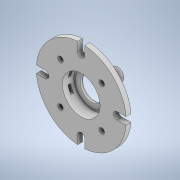
# Autodesk Inventor part: součást 4
Saved by Autodesk Inventor 2022 (Build 260153000, 153)
## iProperties
Created: 2022-03-28
Part Number: součást 4
Material: Všeobecné
Document SubType Name: Modeling
Designer: 27262
Density: 1 g/cm^3
Appearance: Výchozí
Author: 27262
Autodesk Inventor part; units mm, degrees
ref_plane "YZ Plane" through (0, 0, 0) normal (1, 0, 0) x (0, 1, 0)
ref_plane "XZ Plane" through (0, 0, 0) normal (0, 1, 0) x (-1, 0, 0)
ref_plane "XY Plane" through (0, 0, 0) normal (0, 0, 1) x (1, 0, 0)
sketch "Náčrt1" plane through (0, 0, 0) normal (1, 0, 0) x (0, 1, 0)
  line L0 (42, 0) -> (100, 0)
  line L1 (100, 0) -> (100, -11)
  line L2 (100, -11) -> (52, -11)
  line L3 (52, -11) -> (52, -39)
  line L4 (52, -39) -> (42.5, -39)
  line L5 (42.5, -39) -> (42.5, -30)
  line L6 (42.5, -30) -> (26.7321, -30)
  line L7 (26.7321, -30) -> (25, -27)
  line L8 (25, -27) -> (25, -23)
  line L9 (25, -23) -> (36, -23)
  line L10 (36, -23) -> (36, -25.5)
  line L11 (36, -25.5) -> (42, -25.5)
  line L12 (42, -25.5) -> (42, 0)
  line L13 (0, 0) -> (0, -39) construction
  dimension "d0" = 200
  dimension "d1" = 50
  dimension "d2" = 72
  dimension "d3" = 84
  dimension "d4" = 85
  dimension "d5" = 104
  dimension "d6" = 39
  dimension "d7" = 11
  dimension "d8" = 30
  dimension "d9" = 25.5
  dimension "d10" = 23
  dimension "d11" = 4
  dimension "d12" = 30
  constraints: 28 end point, 9 perpendicular, 2 horizontal alignment, 2 vertical, 1 horizontal, 1 parallel
  measures "d0" diameter of L1 L13
  measures "d1" diameter of L8 L13
  measures "d2" diameter of L10 L13
  measures "d3" diameter of L12 L13
  measures "d4" diameter of L5 L13
  measures "d5" diameter of L3 L13
  measures "d6" distance between parallel lines of L0 L4
  measures "d7" distance of L0.end L1.end
  measures "d8" distance between parallel lines of L0 L6
  measures "d9" distance between parallel lines of L0 L11
  measures "d10" distance between parallel lines of L0 L9
  measures "d11" distance of L7.end L8.end
  measures "d12" angle of L7 L8
revolve "Rotace1" add sketch "Náčrt1" angle 360 about axis through (0, 0, 0) along (0, 0, -1)
sketch "Náčrt2" plane through (0, 0, -11) normal (0, 0, -1) x (-1, 0, 0)
  circle A0 centre (0, 0) radius 100 projected
  line L0 (-100, 0) -> (-80, 0) construction
  line L1 (-100, -8) -> (-80, -8)
  line L2 (-80, 8) -> (-100, 8)
  arc A1 (-100, 8) -> (-100, -8) centre (-100, 0) ccw
  arc A2 (-80, -8) -> (-80, 8) centre (-80, 0) ccw
  circle A3 centre (0, 0) radius 52 projected
  line L3 (8, -100) -> (8, -80)
  arc A4 (-8, -100) -> (8, -100) centre (0, -100) ccw
  line L4 (-8, -80) -> (-8, -100)
  arc A5 (8, -80) -> (-8, -80) centre (0, -80) ccw
  line L5 (100, 8) -> (80, 8)
  arc A6 (100, -8) -> (100, 8) centre (100, 0) ccw
  line L6 (80, -8) -> (100, -8)
  arc A7 (80, 8) -> (80, -8) centre (80, 0) ccw
  line L7 (-8, 100) -> (-8, 80)
  arc A8 (8, 100) -> (-8, 100) centre (0, 100) ccw
  line L8 (8, 80) -> (8, 100)
  arc A9 (-8, 80) -> (8, 80) centre (0, 80) ccw
  point P0 (-90, 0)
  dimension "d14" = 16
  dimension "d15" = 80
  dimension "d18" = 360
  constraints: 20 end point, 16 point on circle, 8 centre point, 4 tangent, 2 horizontal alignment, 1 horizontal, 1 midpoint, 1 parallel, 42 other
  measures "d14" diameter of A2
  measures "d15" distance of A3.centre L0.end
extrude "Vysunutí1" cut sketch "Náčrt2" against normal through all contours A0 L6 A7 L5 | A0 L5 A6 L6 | L8 A9 L7 A0 | A0 L7 A8 L8 | L3 A4 L4 A0 | A0 L4 A5 L3 | L2 A2 L1 A0 | A0 L1 A1 L2
sketch "Náčrt3" plane through (0, -80, -11) normal (0, 0, -1) x (-1, 0, 0)
  arc A0 (-80, 72) -> (-80, 88) centre (-80, 80) ccw projected
  line L0 (-80, 80) -> (0, 80) construction
  line L1 (0, 80) -> (-45.9619, 34.0381) construction
  line L2 (-45.3114, 54.4876) -> (-55.8614, 43.9376)
  line L3 (-36.0624, 24.1386) -> (-25.5124, 34.6886)
  line L4 (-21.0972, 78.7018) -> (-39.3358, 20.8652) construction
  line L5 (-59.1348, 40.6642) -> (-1.2982, 58.9028) construction
  arc A1 (-55.8614, 43.9376) -> (-36.0624, 24.1386) centre (-45.9619, 34.0381) ccw
  arc A2 (-55.8614, 43.9376) -> (-36.0624, 24.1386) centre (-45.9619, 34.0381) ccw
  circle A3 centre (0, 80) radius 52 projected
  line L6 (55.8614, 43.9376) -> (45.3114, 54.4876)
  arc A4 (36.0624, 24.1386) -> (55.8614, 43.9376) centre (45.9619, 34.0381) ccw
  line L7 (25.5124, 34.6886) -> (36.0624, 24.1386)
  line L8 (36.0624, 135.8614) -> (25.5124, 125.3114)
  arc A5 (55.8614, 116.0624) -> (36.0624, 135.8614) centre (45.9619, 125.9619) ccw
  line L9 (45.3114, 105.5124) -> (55.8614, 116.0624)
  line L10 (-55.8614, 116.0624) -> (-45.3114, 105.5124)
  arc A6 (-36.0624, 135.8614) -> (-55.8614, 116.0624) centre (-45.9619, 125.9619) ccw
  line L11 (-25.5124, 125.3114) -> (-36.0624, 135.8614)
  point P0 (-30.2165, 49.7835)
  dimension "d22" = 65
  dimension "d23" = 45
  dimension "d26" = 14
  dimension "d29" = 360
  constraints: 24 end point, 12 point on circle, 5 centre point, 2 midpoint, 2 parallel, 2 tangent, 1 coincident, 1 horizontal, 1 point on line, 33 other
  measures "d22" distance of L0.end L1.end
  measures "d23" angle of L0 L1
  measures "d26" radius of A1
extrude "Vysunutí2" add sketch "Náčrt3" along normal blind 24 contours A3 L3 A1 L2 | L10 A6 L11 A3 | A3 L6 A4 L7 | L8 A5 L9 A3
sketch "Náčrt4" plane through (0, -80, -35) normal (0, 0, -1) x (-1, 0, 0)
  arc A0 (-36.0624, 135.8614) -> (-55.8614, 116.0624) centre (-45.9619, 125.9619) ccw projected
  arc A1 (-55.8614, 43.9376) -> (-36.0624, 24.1386) centre (-45.9619, 34.0381) ccw projected
  arc A2 (36.0624, 24.1386) -> (55.8614, 43.9376) centre (45.9619, 34.0381) ccw projected
  arc A3 (55.8614, 116.0624) -> (36.0624, 135.8614) centre (45.9619, 125.9619) ccw projected
  point P0 (0, 80)
  constraints: 4 coincident
hole "Díra1" at (-45.9619, 45.9619, -35) at (45.9619, 45.9619, -35) at (45.9619, -45.9619, -35) at (-45.9619, -45.9619, -35) direction (0, 0, 1) diameter 12 depth 50 tip angle 118
sketch "Náčrt5" plane through (0, 0, 0) normal (1, 0, 0) x (0, 1, 0)
  line L0 (0, 0) -> (0, -39)
  line L1 (-52, -39) -> (52, -39) projected
  line L2 (23, -18) -> (7, -18)
  line L3 (7, -18) -> (7, -12)
  line L4 (7, -12) -> (23, -12)
  line L5 (23, -12) -> (23, -18)
  line L6 (8, 0) -> (99.6795, 0) projected
  line L7 (-23, -18) -> (-7, -18)
  line L8 (-7, -18) -> (-7, -12)
  line L9 (-7, -12) -> (-23, -12)
  line L10 (-23, -12) -> (-23, -18)
  dimension "d40" = 14
  dimension "d41" = 16
  dimension "d42" = 6
  dimension "d43" = 12
  constraints: 18 end point, 4 symmetric about line, 2 parallel, 1 horizontal, 1 midpoint, 1 perpendicular
  measures "d40" diameter of L3 L0
  measures "d41" distance of L3.end L4.end
  measures "d42" distance of L4.end L2.start
  measures "d43" distance between parallel lines of L6 L4
extrude "Vysunutí3" cut sketch "Náčrt5" along normal through all both and the other way through all
